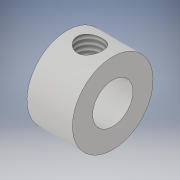
# Autodesk Inventor part: Collar
Saved by Autodesk Inventor 2017 (Build 210142000, 142)
## iProperties
Created: 2018-04-18
Part Number: Collar
Material: Generic
Document SubType Name: Modeling
Designer: User
Density: 1 g/cm^3
Appearance: Default
Author: User
Autodesk Inventor part; units mm, degrees
ref_plane "YZ Plane" through (0, 0, 0) normal (1, 0, 0) x (0, 1, 0)
ref_plane "XZ Plane" through (0, 0, 0) normal (0, 1, 0) x (-1, 0, 0)
ref_plane "XY Plane" through (0, 0, 0) normal (0, 0, 1) x (1, 0, 0)
sketch "Sketch2" plane through (0, 0, 0) normal (0, 0, 1) x (1, 0, 0)
  line L0 (0, 0) -> (7.1755, 0)
  line L1 (0, 6.35) -> (7.1755, 6.35)
  line L2 (7.1755, 6.35) -> (7.1755, 3.175)
  line L3 (7.1755, 3.175) -> (0, 3.175)
  line L4 (0, 3.175) -> (0, 6.35)
  point P0 (3.5877, 6.35)
  dimension "d8" = 7.1755
  dimension "d9" = 3.175
  dimension "d10" = 7.1755
  dimension "d11" = 3.175
  constraints: 10 end point, 2 horizontal, 2 parallel, 1 midpoint, 1 perpendicular
  measures "d8" distance of L0.start L0.end
  measures "d9" distance of L1.end L2.end
  measures "d10" distance of L1.start L1.end
  measures "d11" distance between parallel lines of L0 L3
revolve "Revolution1" add sketch "Sketch2" angle 360 about axis through (0, 0, 0) along (1, 0, 0)
ref_plane "Work Plane1" through (3.5877, 6.35, 0) normal (0, 1, 0) x (-1, 0, 0)
sketch "Sketch3" plane through (3.5877, 6.35, 0) normal (0, 1, 0) x (-1, 0, 0)
  point P0 (3.5877, 0)
  point P1 (0, 0)
hole "Hole1" at (3.5877, 6.35, 0) direction (0, -1, 0) diameter 3.9624 depth 3.175 tip angle 118 thread size "10-32 UNF" class "2B" standard "ANSI Unified Screw Threads"
equation "\"d10\" = d8"
body "Solid2"
